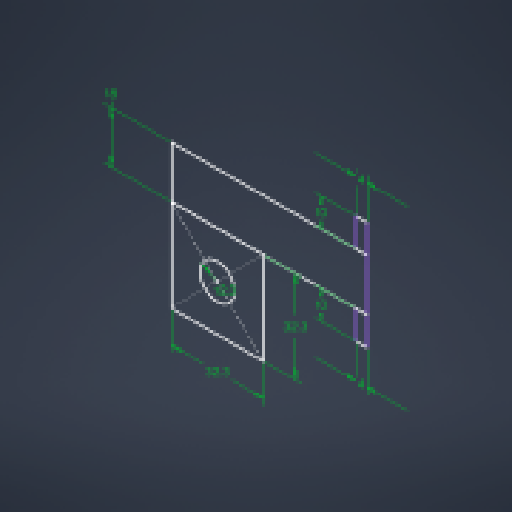
# Autodesk Inventor part: Board-Stand-Center
Saved by Autodesk Inventor 2025 (Build 290162010, 162A)
## iProperties
Created: 2025-12-06
Part Number: Board-Stand-Center
Material: Generic
Document SubType Name: Modeling
Designer: FizzyApple12
Density: 1 g/cm^3
Appearance: Default
Author: FizzyApple12
Autodesk Inventor part; units mm, degrees
ref_plane "YZ Plane" through (0, 0, 0) normal (1, 0, 0) x (0, 1, 0)
ref_plane "XZ Plane" through (0, 0, 0) normal (0, 1, 0) x (-1, 0, 0)
ref_plane "XY Plane" through (0, 0, 0) normal (0, 0, 1) x (1, 0, 0)
sketch "Sketch1" plane through (0, 0, 0) normal (0, 0, 1) x (1, 0, 0)
  line L0 (-16.15, 16.15) -> (16.15, 16.15)
  line L1 (16.15, 16.15) -> (16.15, -16.15)
  line L2 (16.15, -16.15) -> (-16.15, -16.15)
  line L3 (-16.15, -16.15) -> (-16.15, 16.15)
  line L4 (-16.15, 16.15) -> (16.15, -16.15) construction
  line L5 (16.15, 16.15) -> (-16.15, -16.15)
  circle A0 centre (0, 0) radius 6.15
  line L6 (-16.15, 16.15) -> (48, 16.15)
  line L7 (48, 16.15) -> (48, 34.15)
  line L8 (48, 34.15) -> (-16.15, 34.15)
  line L9 (-16.15, 34.15) -> (-16.15, 16.15)
  line L10 (48, 16.15) -> (44, 16.15)
  line L11 (44, 16.15) -> (44, 6.15)
  line L12 (44, 6.15) -> (48, 6.15)
  line L13 (48, 6.15) -> (48, 16.15)
  line L14 (48, 34.15) -> (44, 34.15)
  line L15 (44, 34.15) -> (44, 44.15)
  line L16 (44, 44.15) -> (48, 44.15)
  line L17 (48, 44.15) -> (48, 34.15)
  point P0 (-4.3487, -4.3487)
  point P1 (4.3487, 4.3487)
  point P2 (44, 16.15)
  dimension "d0" = 32.3
  dimension "d1" = 32.3
  dimension "d2" = 12.3
  dimension "d3" = 18
  dimension "d4" = 4
  dimension "d5" = 10
  dimension "d6" = 4
  dimension "d7" = 10
  dimension "d29" = 64.15
  constraints: 36 end point, 8 parallel, 4 horizontal, 4 perpendicular, 2 midpoint, 1 centre point, 1 coincident
  measures "d0" distance of L1.end L2.end
  measures "d1" distance of L0.end L1.end
  measures "d2" diameter of A0
  measures "d3" distance between parallel lines of L8 L6
  measures "d4" distance of L12.end L11.end
  measures "d5" distance of L11.end L10.end
  measures "d6" distance of L15.end L16.end
  measures "d7" distance of L14.end L15.end
  measures "d29" distance between parallel lines of L7 L9
extrude "Extrusion1" add sketch "Sketch1" along normal blind 6.5 contours L9 L8 L7 L6 L0 | L0 L5 A0 L3 | L6 L13 L12 L11 | L15 L16 L17 L8
sketch "Sketch2" plane through (44, 6.15, 0) normal (-1, 0, 0) x (0, 0, 1)
  line L0 (0, 38) -> (0, 28) construction
  line L1 (0, 28) -> (6.5, 28) construction
  line L2 (6.5, 38) -> (6.5, 28) construction
  line L3 (0, 38) -> (6.5, 38) construction
  line L4 (0, 10) -> (0, 0) construction
  line L5 (0, 0) -> (6.5, 0) construction
  line L6 (6.5, 10) -> (6.5, 0) construction
  line L7 (0, 10) -> (6.5, 10) construction
  line L8 (0, 0) -> (6.5, 10) construction
  line L9 (0, 38) -> (6.5, 28) construction
  point P0 (0, -6.15)
  point P1 (3.25, 33)
  point P2 (3.25, 5)
  constraints: 4 end point, 2 midpoint
hole "Hole1" at (44, 39.15, 3.25) at (44, 11.15, 3.25) direction (1, 0, 0) diameter 3.4 end through all clearance for "Socket Head Cap Screw" size "M3" standard "Ansi Metric M Profile"
sketch "Sketch3" plane through (-4.3487, -4.3487, 6.5) normal (0.7071068, -0.7071068, 0) x (-0.7071068, -0.7071068, 0)
  line L0 (0, 6.5) -> (0, 0) construction
  line L1 (0, 3.25) -> (7.85, 3.25) construction
  line L2 (-12.3, 6.5) -> (-12.3, 0) construction
  line L3 (-12.3, 3.25) -> (-20.15, 3.25) construction
  point P0 (-6.15, 6.5)
  dimension "d17" = 28
  constraints: 4 end point, 2 coincident, 2 horizontal, 2 midpoint, 1 collinear
  measures "d17" distance of L3.end L1.end
hole "Hole2" at (9.8995, 9.8995, 3.25) at (-9.8995, -9.8995, 3.25) direction (-0.7071068, 0.7071068, 0) diameter 4.5 depth 6
fillet "Fillet1" radius 1 5 edges at (-16.15, 34.15, 3.25) (-16.15, -16.15, 3.25) (16.15, 16.15, 3.25) (44, 16.15, 3.25) (44, 34.15, 3.25)
chamfer "Chamfer1" distance 0.25 angle 45 44 edges at (4.3487, 4.3487, 3.25) (-4.3487, -4.3487, 3.25) (-9.3958, -9.3958, 0) (-15.5327, -14.6597, 0) (-16.15, 9.7071, 0) (-15.8571, 33.8571, 0) (13.925, 34.15, 0) (43.7071, 34.4429, 0) (44, 39.65, 0) (-9.3958, -9.3958, 6.5) (-15.5327, -14.6597, 6.5) (-16.15, 9.7071, 6.5) (-15.8571, 33.8571, 6.5) (13.925, 34.15, 6.5) (43.7071, 34.4429, 6.5) (44, 39.65, 6.5) (-4.3487, 4.3487, 0) (-4.3487, 4.3487, 6.5) (10.1029, 10.1029, 0) (16.1815, 16.0739, 0) (29.7821, 16.15, 0) (43.7071, 15.8571, 0) (44, 10.65, 0) (10.1029, 10.1029, 6.5) (16.1815, 16.0739, 6.5) (29.7821, 16.15, 6.5) (43.7071, 15.8571, 6.5) (44, 10.65, 6.5) (44, 6.15, 3.25) (48, 6.15, 3.25) (46, 6.15, 6.5) (46, 6.15, 0) (44, 11.15, 1.55) (48, 11.15, 1.55) (48, 25.15, 6.5) (44, 39.15, 1.55) (44, 44.15, 3.25) (48, 44.15, 3.25) (46, 44.15, 0) (48, 25.15, 0) (46, 44.15, 6.5) (48, 39.15, 1.55) (-9.8995, -9.8995, 5.5) (9.8995, 9.8995, 5.5)
body "Solid1"
